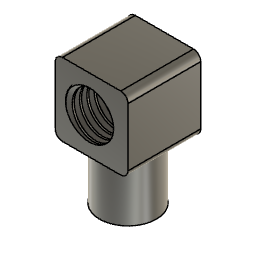
Mini soporte (Autodesk Fusion 360 design; units mm, degrees)
Autodesk Fusion 360 part; units mm, degrees
note: some values were not read from the file. Chosen so that the rebuilt part matches the saved one: which face or edge a step refers to.
sketch "Sketch1" plane through (0, 0, 0) normal (0, 0, 1) x (1, 0, 0)
  circle A0 centre (0, 0) radius 3.9
  dimension "d1" = 7.8
  constraint coincident A0.centre origin
  measures "d1" diameter of A0
extrude "Extrude1" add sketch "Sketch1" along normal blind 7.8
sketch "Sketch2" plane through (0, 0, 7.8) normal (0, 0, 1) x (-1, 0, 0)
  circle A0 centre (0, 0) radius 3.9
  line L0 (-5, 5) -> (5, 5)
  line L1 (5, 5) -> (5, -5)
  line L2 (5, -5) -> (-5, -5)
  line L3 (-5, -5) -> (-5, 5)
  line L4 (-5, 5) -> (5, -5) construction
  line L5 (5, 5) -> (-5, -5) construction
  dimension "d4" = 10
  dimension "d12" = 10
  constraint horizontal L0
  constraint perpendicular L0 L1
  constraint parallel L0 L2
  constraint parallel L1 L3
  constraint coincident L4 A0.centre
  constraint coincident L5 A0.centre
  constraint coincident A0.centre origin
  measures "d4" distance of L1 L3
  measures "d12" distance of L0.start L2.end
extrude "Extrude2" add sketch "Sketch2" along normal blind 10 contours A0 | L0 L1 L2 L3
sketch "Sketch3" plane through (0, -5, 0) normal (0, -1, 0) x (1, 0, 0)
  line L0 (-5, 7.8) -> (5, 7.8)
  line L1 (5, 7.8) -> (5, 17.8)
  line L2 (5, 17.8) -> (-5, 17.8)
  line L3 (-5, 17.8) -> (-5, 7.8)
  line L4 (0, 17.8) -> (0, 7.8) construction
  line L5 (-5, 12.8) -> (5, 12.8) construction
  point P0 (0, 12.8)
  constraint midpoint L2 L4.start
  constraint midpoint L0 L4.end
  constraint midpoint L3 L5.start
  constraint midpoint L1 L5.end
  constraint midpoint L4 P0
hole "Hole1" at (0, -5, 12.8) direction (0, 1, 0) diameter 6.036 depth 18 tip angle 118
thread "Thread1" "ISO Metric profile 7.0 M7x1 6H" major diameter 7.1472 minor diameter 6.0355 pitch 1 angle 60 modelled right hand crest width 0.2748 on face at (0.1504, -1.6667, 9.7858) crest through (0, -4.75, 9.7823)
fillet "Fillet1" radius 1 4 edges at (5, 0, 7.8) (5, 0, 17.8) (-5, 0, 17.8) (-5, 0, 7.8)
